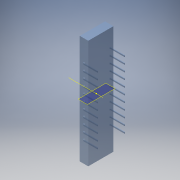
# Autodesk Inventor part: TCD1304AP
Saved by Autodesk Inventor 2017 (Build 210142000, 142)
## iProperties
Created: 2017-01-24
Part Number: TCD1304AP
Material: Glass
Document SubType Name: Modeling
Designer: vmigu
Density: 2.18 g/cm^3
Appearance: Magenta
Author: vmigu
Autodesk Inventor part; units mm, degrees
ref_plane "YZ Plane" through (0, 0, 0) normal (1, 0, 0) x (0, 1, 0)
ref_plane "XZ Plane" through (0, 0, 0) normal (0, 1, 0) x (-1, 0, 0)
ref_plane "XY Plane" through (0, 0, 0) normal (0, 0, 1) x (1, 0, 0)
sketch "Sketch1" plane through (0, 0, 0) normal (1, 0, 0) x (0, 1, 0)
  line L0 (4.825, 20.8) -> (-4.825, 20.8)
  line L1 (-4.825, 20.8) -> (-4.825, -20.8)
  line L2 (-4.825, -20.8) -> (4.825, -20.8)
  line L3 (4.825, -20.8) -> (4.825, 20.8)
  line L4 (4.825, 20.8) -> (-4.825, -20.8) construction
  line L5 (-4.825, 20.8) -> (4.825, -20.8) construction
  point P0 (0, 0)
  dimension "d0" = 9.65
  dimension "d1" = 41.6
  constraints: 12 end point, 2 midpoint, 2 parallel, 1 horizontal, 1 perpendicular
  measures "d0" distance of L2.end L1.end
  measures "d1" distance of L1.end L0.end
extrude "Extrusion1" add sketch "Sketch1" along normal blind 3.22
sketch "Sketch2" plane through (0, 0, 0) normal (-1, 0, 0) x (0, 0, 1)
  line L0 (-14.55, 0.5) -> (14.55, 0.5)
  line L1 (14.55, 0.5) -> (14.55, -0.5)
  line L2 (14.55, -0.5) -> (-14.55, -0.5)
  line L3 (-14.55, -0.5) -> (-14.55, 0.5)
  line L4 (-14.55, 0.5) -> (14.55, -0.5) construction
  line L5 (14.55, 0.5) -> (-14.55, -0.5) construction
  point P0 (0, 0)
  dimension "d4" = 29.1
  dimension "d5" = 1
  constraints: 12 end point, 2 midpoint, 2 parallel, 1 horizontal, 1 perpendicular
  measures "d4" distance of L1.end L2.end
  measures "d5" distance of L0.end L1.end
extrude "Extrusion2" cut sketch "Sketch2" against normal blind 1.52
chamfer "Chamfer1" distance 1.52 angle 45 4 edges at (0, 0.5, 0) (0, 0, -14.55) (0, -0.5, 0) (0, 0, 14.55)
sketch "Sketch3" plane through (1.52, 0, 0) normal (-1, 0, 0) x (0, 0, 1)
  point P0 (0, 0)
ref_plane "Work Plane1" through (1.52, -0.5, 0) normal (0, 0, -1) x (-1, 0, 0)
sketch "Sketch4" plane through (1.52, -0.5, 0) normal (0, 0, -1) x (-1, 0, 0)
  line L0 (1.52, 5.325) -> (-1.7, 5.325) projected
  line L1 (1.52, 0.5) -> (-1.7, 0.5) construction
  line L2 (-1.7, 5.325) -> (-1.7, -4.325) projected
  arc A0 (-0.215, 5.325) -> (-0.44, 5.55) centre (-0.44, 5.325) ccw
  arc A1 (0.035, 5.325) -> (-0.44, 5.8) centre (-0.44, 5.325) ccw
  line L3 (-0.44, 5.8) -> (-5.7, 5.8)
  line L4 (-5.7, 5.8) -> (-5.7, 5.55)
  line L5 (-5.7, 5.55) -> (-0.44, 5.55)
  line L6 (-0.215, 5.325) -> (0.035, 5.325)
  arc A2 (-0.44, -4.55) -> (-0.215, -4.325) centre (-0.44, -4.325) ccw
  arc A3 (-0.44, -4.8) -> (0.035, -4.325) centre (-0.44, -4.325) ccw
  line L7 (-0.44, -4.8) -> (-5.7, -4.8)
  line L8 (-5.7, -4.8) -> (-5.7, -4.55)
  line L9 (-5.7, -4.55) -> (-0.44, -4.55)
  line L10 (-0.215, -4.325) -> (0.035, -4.325)
  point P0 (-0.09, 5.325)
  point P1 (-0.09, -4.325)
  dimension "d11" = 0.25
  dimension "d13" = 4
  dimension "d15" = 10.1
  dimension "d16" = 0.25
  constraints: 18 end point, 9 symmetric about line, 8 point on circle, 4 centre point, 3 midpoint, 2 perpendicular, 2 point on line, 2 tangent, 1 collinear, 1 concentric, 1 horizontal, 2 other
  measures "d11" distance of L6.end L6.start
  measures "d13" distance between parallel lines of L2 L4
  measures "d15" diameter of L5 L1
  measures "d16" distance of L3.end L4.end
extrude "Extrusion3" add sketch "Sketch4" along normal mid plane 0.47
pattern_linear "Rectangular Pattern1" count 11 spacing 2.54 along (0, 0, 1) of "Extrusion3" first direction both ways yes
ref_plane "Work Plane2" through (1.52, 0, 0) normal (0, 1, 0) x (1, 0, 0)
sketch "Sketch5" plane through (0, 0, 0) normal (-1, 0, 0) x (0, 0, 1)
  line L0 (-20.8, -4.825) -> (-20.8, 4.825) projected
  circle A0 centre (-20.8, 0) radius 1.5
  point P0 (0, 0)
  dimension "d22" = 3
  constraints: 1 centre point, 1 midpoint
  measures "d22" diameter of A0
extrude "Extrusion4" cut sketch "Sketch5" against normal through all
equation "\"d16\" = d11"
body "Solid1"
